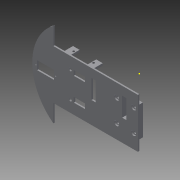
# Autodesk Inventor part: chasis_robot_kedama_rev7
Saved by Autodesk Inventor 2015 (Build 190159000, 159)
## iProperties
Created: 2021-04-17
Part Number: chasis_robot_kedama_rev7
Material: Generic
Document SubType Name: Modeling
Designer: 34617
Density: 1 g/cm^3
Appearance: Default
Author: 34617
Autodesk Inventor part; units mm, degrees
ref_plane "YZ Plane" through (0, 0, 0) normal (1, 0, 0) x (0, 1, 0)
ref_plane "XZ Plane" through (0, 0, 0) normal (0, 1, 0) x (-1, 0, 0)
ref_plane "XY Plane" through (0, 0, 0) normal (0, 0, 1) x (1, 0, 0)
sketch "Sketch1" plane through (0, 0, 0) normal (0, 1, 0) x (-1, 0, 0)
  line L0 (0, -60) -> (150, -60) construction
  line L1 (75, 0) -> (75, -120) construction
  line L2 (150, 0) -> (120, 0) construction
  line L3 (120, 0) -> (120, -120) construction
  line L4 (120, -120) -> (150, -120) construction
  arc A0 (120, -120) -> (120, 0) centre (75, -60) ccw
  line L5 (0, -25) -> (120, -25)
  line L6 (120, -25) -> (120, 0)
  line L7 (0, -95) -> (120, -95)
  line L8 (120, -95) -> (120, -120)
  line L9 (0, -25) -> (0, -95)
  point P0 (0, 0)
  dimension "d2" = 30
  dimension "d4" = 120
  dimension "d6" = 120
  dimension "d7" = 75
  dimension "d8" = 60
  dimension "d9" = 95
  dimension "d10" = 25
  dimension "d11" = 0
  dimension "d12" = 120
  dimension "d13" = 30
  dimension "d14" = 30
  dimension "d15" = 0
  dimension "d16" = 120
  constraints: 20 end point, 6 parallel, 2 point on circle, 1 centre point, 1 horizontal, 1 midpoint, 1 perpendicular, 1 tangent, 1 vertical
  measures "d2" distance of L4.end L3.end
  measures "d4" distance of L5.start L5.end
  measures "d6" distance of L7.start L7.end
  measures "d7" radius of A0
  measures "d8" distance between parallel lines of L2 L0
  measures "d9" distance between parallel lines of L2 L7
  measures "d10" distance between parallel lines of L2 L5
  measures "d11" distance from line of point (0, 0) L2
  measures "d12" distance from line of point (0, 0) L6
  measures "d13" distance from line of L2.start L6
  measures "d14" distance from line of L0.end L6
  measures "d15" distance from line of L1.start L2
  measures "d16" distance from line of L0.start L6
extrude "Extrusion1" add sketch "Sketch1" along normal blind 2
sketch "Sketch2" plane through (0, 2, 0) normal (0, 1, 0) x (1, 0, 0)
  line L0 (0, 25) -> (0, 95) construction
  line L1 (0, 60) -> (-150, 60) construction
  arc A0 (-120, 120) -> (-120, 0) centre (-75, 60) ccw construction
  line L2 (-117.4507, 52.0399) -> (-117.4507, 68.4308) construction
  line L3 (-114.9012, 60) -> (-114.9012, 66.1) construction
  line L4 (-114.9012, 66.1) -> (-147.0012, 66.1) construction
  line L5 (-147.0012, 66.1) -> (-147.0012, 53.9) construction
  line L6 (-114.9012, 53.9) -> (-114.9012, 60) construction
  line L7 (-147.0012, 60) -> (-147.0012, 62) construction
  line L8 (-147.0012, 62) -> (-143.0012, 62) construction
  line L9 (-143.0012, 62) -> (-143.0012, 58) construction
  line L10 (-143.0012, 58) -> (-147.0012, 58) construction
  line L11 (-147.0012, 60) -> (-147.0012, 58) construction
  line L12 (-143.0012, 58) -> (-147.0012, 62) construction
  line L13 (-143.0012, 62) -> (-147.0012, 58) construction
  circle A1 centre (-145.0012, 60) radius 1
  line L14 (-114.9012, 60) -> (-114.9012, 62) construction
  line L15 (-114.9012, 62) -> (-118.9012, 62) construction
  line L16 (-118.9012, 62) -> (-118.9012, 58) construction
  line L17 (-118.9012, 58) -> (-114.9012, 58) construction
  line L18 (-118.9012, 62) -> (-114.9012, 62) construction
  line L19 (-114.9012, 58) -> (-114.9012, 62) construction
  line L20 (-114.9012, 58) -> (-118.9012, 62) construction
  line L21 (-114.9012, 62) -> (-118.9012, 58) construction
  circle A2 centre (-116.9012, 60) radius 1
  line L22 (-145.0012, 60) -> (-116.9012, 60) construction
  line L23 (-143.0012, 66.0861) -> (-118.9012, 66.1)
  line L24 (-118.9012, 66.1) -> (-118.8942, 54)
  line L25 (-118.8942, 54) -> (-142.9942, 54)
  line L26 (-142.9942, 54) -> (-142.9942, 66.1)
  point P0 (0, 0)
  dimension "d22" = 117.4507
  dimension "d103" = 32.1
  dimension "d104" = 12.2
  dimension "d105" = 32.1
  dimension "d106" = 2
  dimension "d107" = 4
  dimension "d108" = 4
  dimension "d109" = 2
  dimension "d113" = 2
  dimension "d114" = 28.1
  dimension "d116" = 114.9012
  dimension "d117" = 2
  dimension "d118" = 118.9012
  dimension "d119" = 8.4308
  dimension "d120" = 7.9601
  dimension "d124" = 24.1
  dimension "d125" = 12.1
  dimension "d127" = 0.033
  dimension "d128" = 24.1
  dimension "d129" = 12.1
  constraints: 52 end point, 11 perpendicular, 11 point on line, 4 collinear, 4 midpoint, 2 centre point, 2 parallel, 1 horizontal, 1 point on circle
  measures "d22" distance between parallel lines of L2 L0
  measures "d103" distance of L3.end L4.end
  measures "d104" distance of L4.end L5.end
  measures "d105" distance of L5.end L6.start
  measures "d106" distance of L7.start L7.end
  measures "d107" distance of L7.end L8.end
  measures "d108" distance of L8.end L9.end
  measures "d109" diameter of A1
  measures "d113" diameter of A2
  measures "d114" distance of L22.start L22.end
  measures "d116" distance between parallel lines of L3 L0
  measures "d117" distance between parallel lines of L1 L15
  measures "d118" distance from line of L0.end L16
  measures "d119" distance from line of L2.end L1
  measures "d120" distance from line of L2.start L1
  measures "d124" distance of L23.start L23.end
  measures "d125" distance of L23.end L24.end
  measures "d127" angle of L24 L0
  measures "d128" distance of L24.end L25.end
  measures "d129" distance of L25.end L26.end
sketch "Sketch3" plane through (0, 2, 0) normal (0, 1, 0) x (1, 0, 0)
  line L0 (0, 25) -> (0, 95) construction
  line L1 (0, 60) -> (-150, 60) construction
  circle A0 centre (-30.0032, 43.5012) radius 2
  circle A1 centre (-30.0032, 75.0012) radius 2
  circle A2 centre (-6.0032, 75.0012) radius 2
  circle A3 centre (-6.0032, 43.5012) radius 2
  line L2 (-30.0032, 43.5012) -> (-30.0032, 75.0012) construction
  line L3 (-6.0032, 43.5012) -> (-6.0032, 75.0012) construction
  line L4 (-30.0032, 43.5012) -> (-6.0032, 43.5012) construction
  line L5 (-30.0032, 75.0012) -> (-6.0032, 75.0012) construction
  point P0 (0, 0)
  dimension "d29" = 150
  dimension "d36" = 4
  dimension "d37" = 4
  dimension "d41" = 31.5
  dimension "d42" = 31.5
  dimension "d43" = 24
  dimension "d44" = 24
  dimension "d45" = 6.0032
  dimension "d46" = 16.4988
  constraints: 10 end point, 4 centre point, 2 equal radius, 2 horizontal, 2 vertical, 1 midpoint
  measures "d29" distance of L1.start L1.end
  measures "d36" diameter of A0
  measures "d37" diameter of A1
  measures "d41" distance of L2.start L2.end
  measures "d42" distance of L3.start L3.end
  measures "d43" distance of L2.start L3.start
  measures "d44" distance of L2.end L3.end
  measures "d45" distance between parallel lines of L0 L3
  measures "d46" distance between parallel lines of L1 L4
extrude "Extrusion3" cut sketch "Sketch3" against normal blind 11
sketch "Sketch4" plane through (0, 2, 0) normal (0, 1, 0) x (1, 0, 0)
  line L0 (0, 95) -> (-120, 95) construction
  line L1 (-120, 25) -> (-50, 25) construction
  line L2 (-50, 25) -> (-50, 95) construction
  line L3 (-50, 95) -> (-120, 95) construction
  line L4 (-120, 95) -> (-120, 25) construction
  line L5 (-120, 95) -> (-50, 95) construction
  line L6 (-50, 95) -> (-50, 85) construction
  line L7 (-120, 85) -> (-120, 95) construction
  line L8 (-50, 25) -> (-50, 35) construction
  line L9 (-120, 35) -> (-120, 25) construction
  line L10 (-120, 30) -> (-50, 30) construction
  line L11 (-75, 80) -> (-91, 80)
  line L12 (-91, 40) -> (-75, 40)
  line L13 (-85, 95) -> (-85, 73) construction
  line L14 (-91, 73) -> (-75, 73)
  line L15 (-75, 73) -> (-75, 80) construction
  line L16 (-91, 80) -> (-91, 73)
  line L17 (-75, 80) -> (-75, 73)
  line L18 (-75, 73) -> (-75, 25) construction
  line L19 (-91, 47) -> (-75, 47)
  line L20 (-91, 47) -> (-91, 40)
  line L21 (-75, 47) -> (-75, 40)
  line L22 (-85, 73) -> (-85, 25) construction
  line L23 (-75, 80) -> (-75, 95) construction
  line L24 (-91, 80) -> (-91, 95) construction
  line L25 (-85, 95) -> (-91, 95)
  line L26 (-91, 95) -> (-91, 92.5)
  line L27 (-91, 92.5) -> (-79, 92.5)
  line L28 (-79, 92.5) -> (-79, 95)
  line L29 (-85, 25) -> (-91, 25)
  line L30 (-120, 25) -> (0, 25) projected
  line L31 (-91, 25) -> (-91, 27.5)
  line L32 (-91, 27.5) -> (-79, 27.5)
  line L33 (-79, 27.5) -> (-79, 25)
  line L34 (-85, 25) -> (-79, 25)
  line L35 (-79, 27.5) -> (-91, 27.5)
  line L36 (-75, 40) -> (-70, 40)
  line L37 (-70, 40) -> (-70, 47)
  line L38 (-70, 47) -> (-75, 47)
  line L39 (-75, 73) -> (-69.9974, 73)
  line L40 (-69.9974, 73) -> (-69.9974, 80)
  line L41 (-69.9974, 80) -> (-75, 80)
  point P0 (0, 0)
  dimension "d49" = 70
  dimension "d51" = 10
  dimension "d52" = 10
  dimension "d70" = 6
  dimension "d71" = 2.5
  dimension "d72" = 12
  dimension "d73" = 6
  dimension "d74" = 2.5
  dimension "d75" = 12
  dimension "d76" = 55
  dimension "d77" = 22
  dimension "d78" = 65
  dimension "d79" = 0
  dimension "d80" = 25
  dimension "d81" = 70
  dimension "d219" = 5
  dimension "d220" = 7
  dimension "d221" = 16
  dimension "d222" = 16
  constraints: 80 end point, 17 perpendicular, 11 parallel, 8 point on line, 4 collinear, 3 horizontal, 3 midpoint, 1 vertical
  measures "d49" distance of L3.end L2.end
  measures "d51" distance of L5.end L6.end
  measures "d52" distance of L8.start L8.end
  measures "d70" distance of L13.start L25.end
  measures "d71" distance of L25.end L26.end
  measures "d72" distance of L26.end L27.end
  measures "d73" distance of L22.end L29.end
  measures "d74" distance of L29.end L31.end
  measures "d75" distance of L31.end L32.end
  measures "d76" distance between parallel lines of L30 L11
  measures "d77" distance between parallel lines of L30 L19
  measures "d78" distance between parallel lines of L10 L0
  measures "d79" distance between parallel lines of L2 L6
  measures "d80" distance between parallel lines of L18 L6
  measures "d81" distance from line of L18.end L0
  measures "d219" distance of L12.end L36.end
  measures "d220" distance of L39.end L40.end
  measures "d221" distance of L12.start L12.end
  measures "d222" distance of L14.start L14.end
extrude "Extrusion5" cut sketch "Sketch4" against normal blind 3 contours L17 L14 L16 L11 | L20 L19 L21 L12
sketch "Sketch5" plane through (0, 2, 0) normal (0, 1, 0) x (1, 0, 0)
  line L0 (-120, 25) -> (0, 25) construction
  line L1 (-85, 25) -> (-85, 95) construction
  line L2 (0, 95) -> (-120, 95) construction
  line L3 (-85, 25) -> (-91, 25)
  line L4 (-85, 25) -> (-79, 25)
  line L5 (-85, 95) -> (-91, 95)
  line L6 (-85, 95) -> (-79, 95)
  line L7 (-85, 28) -> (-101.1, 28)
  line L8 (-85, 28) -> (-68.9, 28)
  line L9 (-85, 92) -> (-101.1, 92)
  line L10 (-85, 92) -> (-68.9, 92)
  line L11 (-68.9, 92) -> (-68.9, 95)
  line L12 (0, 95) -> (-120, 95) projected
  line L13 (-101.1, 92) -> (-101.1, 95)
  line L14 (-68.9, 95) -> (-101.1, 95)
  line L15 (-101.1, 28) -> (-101.1, 25)
  line L16 (-68.9, 25) -> (-101.1, 25)
  line L17 (-68.9, 28) -> (-68.9, 25)
  point P0 (0, 0)
  dimension "d84" = 6
  dimension "d157" = 16.1
  dimension "d158" = 16.1
  dimension "d159" = 16.1
  dimension "d160" = 16.1
  dimension "d169" = 90
  dimension "d170" = 90
  dimension "d171" = 67
  dimension "d172" = 3
  dimension "d173" = 0
  dimension "d174" = 16.1
  dimension "d175" = 68.9
  dimension "d176" = 10.1
  dimension "d177" = 10.1
  dimension "d178" = 22.1
  constraints: 30 end point, 10 point on line, 5 perpendicular, 3 collinear, 2 horizontal, 1 vertical
  measures "d84" distance of L1.start L3.end
  measures "d157" distance of L7.start L7.end
  measures "d158" distance of L7.start L8.end
  measures "d159" distance of L9.start L9.end
  measures "d160" distance of L9.start L10.end
  measures "d169" angle of L9 L11
  measures "d170" angle of L7 L11
  measures "d171" distance between parallel lines of L12 L8
  measures "d172" distance between parallel lines of L10 L2
  measures "d173" distance between parallel lines of L11 L17
  measures "d174" distance between parallel lines of L11 L1
  measures "d175" distance from line of L2.start L11
  measures "d176" distance from line of L6.end L11
  measures "d177" distance from line of L4.end L11
  measures "d178" distance from line of L5.end L11
extrude "Extrusion6" add sketch "Sketch5" along normal blind 12
sketch "Sketch6" plane through (-120, 0, -25) normal (0, 0, 1) x (1, 0, 0)
  line L0 (120, 0) -> (0, 0) construction
  line L1 (18.9, 2) -> (51.1, 2) construction
  line L2 (18.9, 2) -> (18.9, 14) construction
  line L3 (18.9, 8) -> (51.1, 8) construction
  line L4 (51.1, 2) -> (51.1, 14) construction
  line L5 (18.9, 8) -> (19.4, 8) construction
  line L6 (19.4, 8) -> (19.4, 14) construction
  line L7 (19.4, 8) -> (19.4, 2) construction
  line L8 (51.1, 2) -> (18.9, 2) construction
  line L9 (51.1, 8) -> (50.6, 8) construction
  line L10 (50.6, 8) -> (50.6, 14) construction
  line L11 (50.6, 14) -> (50.6, 2) construction
  line L12 (19.4, 8) -> (20.9, 8) construction
  circle A0 centre (20.9, 8) radius 1.5
  line L13 (50.6, 8) -> (49.1, 8) construction
  circle A1 centre (49.1, 8) radius 1.5
  dimension "d162" = 0.5
  dimension "d163" = 0.5
  dimension "d164" = 1.5
  dimension "d165" = 3
  dimension "d166" = 1.5
  dimension "d167" = 3
  dimension "d168" = 32.2
  dimension "d179" = 14
  dimension "d180" = 14
  constraints: 20 end point, 8 point on line, 2 centre point, 2 coincident, 2 midpoint, 2 perpendicular, 1 horizontal
  measures "d162" distance of L3.start L5.end
  measures "d163" distance of L3.end L9.end
  measures "d164" distance of L5.end L12.end
  measures "d165" diameter of A0
  measures "d166" distance of L9.end L13.end
  measures "d167" diameter of A1
  measures "d168" distance of L3.start L3.end
  measures "d179" distance from line of L10.end L0
  measures "d180" distance from line of L6.end L0
extrude "Extrusion7" cut sketch "Sketch6" against normal blind 3
sketch "Sketch7" plane through (0, 0, -95) normal (0, 0, -1) x (-1, 0, 0)
  line L0 (120, 0) -> (0, 0) construction
  line L1 (68.9, 2) -> (101.1, 2) construction
  line L2 (68.9, 2) -> (101.1, 2) construction
  line L3 (68.9, 2) -> (68.9, 14) construction
  line L4 (68.9, 8) -> (101.1, 8) construction
  circle A0 centre (70.9, 8) radius 1.5 projected
  circle A1 centre (70.9, 8) radius 1.5
  circle A2 centre (99.1, 8) radius 1.5 projected
  circle A3 centre (99.1, 8) radius 1.5
  constraints: 4 end point, 2 centre point, 2 coincident, 1 collinear, 1 horizontal, 1 midpoint
extrude "Extrusion8" cut sketch "Sketch7" against normal blind 3
extrude "Extrusion9" cut sketch "Sketch2" against normal blind 3 contours A1 | A2
sketch "Sketch9" plane through (0, 2, 0) normal (0, 1, 0) x (1, 0, 0)
  circle A0 centre (-116.9012, 60) radius 1 construction
  circle A1 centre (-145.0012, 60) radius 1 construction
  line L0 (-116.9012, 60) -> (-145.0012, 60) construction
  line L1 (-145.0012, 60) -> (-150, 60) construction
  arc A2 (-120, 120) -> (-120, 0) centre (-75, 60) ccw construction
  line L2 (-144.0012, 60) -> (-143.0012, 60) construction
  line L3 (-143.0012, 60) -> (-143.0012, 66.1)
  line L4 (-143.0012, 66.1) -> (-119.0012, 66.1)
  line L5 (-119.0012, 66.1) -> (-119.0012, 53.9)
  line L6 (-119.0012, 53.9) -> (-143.0012, 53.9)
  line L7 (-143.0012, 53.9) -> (-143.0012, 60)
  point P0 (0, 0)
  dimension "d130" = 1
  dimension "d131" = 6.1
  dimension "d132" = 24
  dimension "d133" = 12.2
  constraints: 16 end point, 5 perpendicular, 4 point on line, 1 horizontal, 1 horizontal alignment, 1 point on circle, 1 other
  measures "d130" distance of L2.start L2.end
  measures "d131" distance of L2.end L3.end
  measures "d132" distance of L3.end L4.end
  measures "d133" distance of L4.end L5.end
extrude "Extrusion10" cut sketch "Sketch9" against normal blind 2
sketch "Sketch10" plane through (0, 2, 0) normal (0, 1, 0) x (1, 0, 0)
  line L0 (0, 25) -> (0, 95) projected
  line L1 (-34.3549, 37.8531) -> (0, 37.8531)
  line L2 (0, 37.8531) -> (0, 80.7294)
  line L3 (0, 80.7294) -> (-34.3549, 80.7294)
  line L4 (-34.3549, 80.7294) -> (-34.3549, 37.8531)
  circle A0 centre (-30.0032, 43.5012) radius 2 projected
  circle A1 centre (-30.0032, 43.5012) radius 2
  circle A2 centre (-30.0032, 75.0012) radius 2 projected
  circle A3 centre (-30.0032, 75.0012) radius 2
  circle A4 centre (-6.0032, 43.5012) radius 2 projected
  circle A5 centre (-6.0032, 43.5012) radius 2
  circle A6 centre (-6.0032, 75.0012) radius 2.1402
  point P0 (0, 0)
  dimension "d136" = 34.3548
  dimension "d137" = 42.8763
  dimension "d138" = 14.2706
  dimension "d147" = 4.2805
  dimension "d148" = 4
  dimension "d149" = 4
  dimension "d150" = 4
  dimension "d151" = 6.0032
  dimension "d152" = 5.7282
  constraints: 8 end point, 4 centre point, 3 coincident, 2 parallel, 1 horizontal, 1 perpendicular, 1 point on line
  measures "d136" distance between parallel lines of L4 L0
  measures "d137" distance between parallel lines of L3 L1
  measures "d138" distance from line of L0.end L3
  measures "d147" diameter of A6
  measures "d148" diameter of A5
  measures "d149" diameter of A3
  measures "d150" diameter of A1
  measures "d151" distance from line of A6.centre L0
  measures "d152" distance from line of A6.centre L3
extrude "Extrusion11" add sketch "Sketch10" along normal blind 5 contours L1 L4 L3 L0 | A0 | A2 | A4 | A6
sketch "Sketch11" plane through (0, 7, 0) normal (0, 1, 0) x (1, 0, 0)
  circle A0 centre (-30.0032, 43.5012) radius 2 projected
  circle A1 centre (-30.0032, 43.5012) radius 2
  circle A2 centre (-30.0032, 75.0012) radius 2 projected
  circle A3 centre (-30.0032, 75.0012) radius 2
  circle A4 centre (-6.0032, 43.5012) radius 2 projected
  circle A5 centre (-6.0032, 43.5012) radius 2
  circle A6 centre (-6.0032, 75.0012) radius 2 projected
  circle A7 centre (-6.0032, 75.0012) radius 2
  point P0 (0, 0)
  constraints: 4 centre point, 4 coincident
extrude "Extrusion12" cut sketch "Sketch11" against normal blind 11
sketch "Sketch13" plane through (0, 2, 0) normal (0, 1, 0) x (1, 0, 0)
  point P0 (0, 0)
sketch "Sketch14" plane through (0, 2, 0) normal (0, 1, 0) x (1, 0, 0)
  line L0 (-122.4098, 34.6229) -> (-134.4098, 34.6229)
  line L1 (-134.4098, 34.6229) -> (-134.4098, 42.6229)
  line L2 (-134.4098, 42.6229) -> (-122.4098, 42.6229)
  line L3 (-122.4098, 42.6229) -> (-122.4098, 34.6229)
  point P0 (0, 0)
  dimension "d183" = 12
  dimension "d184" = 8
  constraints: 8 end point, 2 parallel, 1 horizontal, 1 perpendicular
  measures "d183" distance of L1.end L2.end
  measures "d184" distance of L0.end L1.end
extrude "Extrusion14" add sketch "Sketch14" along normal blind 0.5
sketch "Sketch16" plane through (0, 2.5, 0) normal (0, 1, 0) x (1, 0, 0)
  line L0 (-130.4881, 40.8759) -> (-125.3198, 40.8759) construction
  line L1 (-125.3198, 40.8759) -> (-125.3198, 24.6109) construction
  line L2 (-125.3198, 24.6109) -> (-130.4881, 24.6109) construction
  line L3 (-130.4881, 24.6109) -> (-130.4881, 40.8759) construction
  line L4 (-123.6414, 30.8759) -> (-125.3675, 30.8759)
  line L5 (-125.3675, 30.8759) -> (-129.0223, 35.5274)
  line L6 (-129.0223, 35.5274) -> (-129.6057, 34.871)
  line L7 (-129.6057, 34.871) -> (-129.6057, 30.8759)
  line L8 (-129.6057, 30.8759) -> (-130.9347, 30.8759)
  line L9 (-130.9347, 30.8759) -> (-130.9347, 40.8759)
  line L10 (-130.9347, 40.8759) -> (-129.6057, 40.8759)
  line L11 (-129.6057, 40.8759) -> (-129.6057, 36.2811)
  line L12 (-129.6057, 36.2811) -> (-125.5052, 40.8759)
  line L13 (-125.5052, 40.8759) -> (-123.8845, 40.8759)
  line L14 (-123.8845, 40.8759) -> (-128.0255, 36.4107)
  line L15 (-128.0255, 36.4107) -> (-123.6414, 30.8759)
  point P0 (0, 0)
  dimension "d270" = 5.1682
  dimension "d271" = 16.265
  dimension "d272" = 125.3198
  dimension "d273" = 40.8759
  constraints: 1 horizontal, 2 other
  measures "d270" distance between parallel lines of L3 L1
  measures "d271" distance between parallel lines of L0 L2
  measures "d272" distance from line of point (0, 0) L1
  measures "d273" distance from line of point (0, 0) L0
extrude "Extrusion15" add sketch "Sketch16" along normal blind 1.5
sketch "Sketch17" plane through (-120, 0, -25) normal (0, 0, 1) x (1, 0, 0)
  line L0 (18.9, 14) -> (51.1, 14) projected
  line L1 (23.2569, 14) -> (46.8571, 14)
  line L2 (46.8571, 14) -> (46.8571, 2)
  line L3 (46.8571, 2) -> (23.2569, 2)
  line L4 (23.2569, 2) -> (23.2569, 14)
  point P0 (120, 0)
  dimension "d189" = 12
  dimension "d190" = 23.6002
  dimension "d191" = 73.1429
  constraints: 8 end point, 2 parallel, 1 horizontal, 1 perpendicular, 1 point on line
  measures "d189" distance of L3.end L1.start
  measures "d190" distance of L2.end L3.end
  measures "d191" distance from line of point (120, 0) L2
extrude "Extrusion16" cut sketch "Sketch17" against normal blind 3
sketch "Sketch18" plane through (-120, 0, -25) normal (0, 0, 1) x (1, 0, 0)
  line L0 (18.9, 2) -> (13.9, 2)
  line L1 (13.9, 2) -> (13.9, 14)
  line L2 (13.9, 14) -> (18.9, 14)
  line L3 (18.9, 14) -> (18.9, 2)
  line L4 (51.1, 2) -> (56.1, 2)
  line L5 (56.1, 2) -> (56.1, 14)
  line L6 (56.1, 14) -> (51.1, 14)
  line L7 (51.1, 14) -> (51.1, 2)
  point P0 (120, 0)
  dimension "d194" = 5
  dimension "d195" = 12
  dimension "d196" = 5
  dimension "d197" = 12
  constraints: 16 end point, 4 parallel, 2 horizontal, 2 perpendicular
  measures "d194" distance of L1.end L2.end
  measures "d195" distance of L0.end L1.end
  measures "d196" distance of L6.end L5.end
  measures "d197" distance of L4.end L5.end
extrude "Extrusion17" add sketch "Sketch18" against normal blind 3
sketch "Sketch19" plane through (0, 0, -95) normal (0, 0, -1) x (-1, 0, 0)
  line L0 (73.1429, 14) -> (96.7431, 14)
  line L1 (96.7431, 14) -> (96.7431, 2)
  line L2 (96.7431, 2) -> (73.1429, 2)
  line L3 (73.1429, 2) -> (73.1429, 14)
  point P0 (0, 0)
  constraints: 8 end point, 2 parallel, 1 horizontal, 1 perpendicular
extrude "Extrusion18" cut sketch "Sketch19" against normal blind 3
sketch "Sketch20" plane through (0, 0, -95) normal (0, 0, -1) x (-1, 0, 0)
  line L0 (68.9, 2) -> (63.9, 2)
  line L1 (63.9, 2) -> (63.9, 14)
  line L2 (63.9, 14) -> (68.9, 14)
  line L3 (68.9, 14) -> (68.9, 2)
  line L4 (101.1, 2) -> (106.1, 2)
  line L5 (106.1, 2) -> (106.1, 14)
  line L6 (106.1, 14) -> (101.1, 14)
  line L7 (101.1, 14) -> (101.1, 2)
  point P0 (0, 0)
  constraints: 16 end point, 4 parallel, 2 horizontal, 2 perpendicular
extrude "Extrusion19" add sketch "Sketch20" against normal blind 3
sketch "Sketch21" plane through (0, 0, 0) normal (0, -1, 0) x (1, 0, 0)
  circle A0 centre (-6.036, -74.9232) radius 3.5
  circle A1 centre (-30.0796, -74.9232) radius 3.5
  circle A2 centre (-30.0796, -43.3906) radius 3.5
  circle A3 centre (-6.036, -43.3906) radius 3.5
  point P0 (0, 0)
  dimension "d204" = 7
  dimension "d205" = 7
  dimension "d206" = 7
  dimension "d207" = 7
  constraints: 4 centre point
  measures "d204" diameter of A0
  measures "d205" diameter of A1
  measures "d206" diameter of A2
  measures "d207" diameter of A3
extrude "Extrusion20" cut sketch "Sketch21" against normal blind 2
sketch "Sketch22" plane through (0, 2, 0) normal (0, 1, 0) x (1, 0, 0)
  line L0 (-78.4615, 36.6997) -> (-113.3615, 36.6997) construction
  line L1 (-113.3615, 36.6997) -> (-113.3615, 83.9997) construction
  line L2 (-113.3615, 83.9997) -> (-78.4615, 83.9997) construction
  line L3 (-78.4615, 83.9997) -> (-78.4615, 36.6997) construction
  line L4 (-78.4615, 60.3497) -> (-113.3615, 60.3497) construction
  circle A0 centre (-95.9115, 41.8497) radius 2
  circle A1 centre (-95.9115, 78.8497) radius 2
  line L5 (-17.2206, 25.8993) -> (-68.7206, 25.8993) construction
  line L6 (-68.7206, 25.8993) -> (-68.7206, 93.3993) construction
  line L7 (-68.7206, 93.3993) -> (-17.2206, 93.3993) construction
  line L8 (-17.2206, 93.3993) -> (-17.2206, 25.8993) construction
  line L9 (-68.7206, 93.3993) -> (-62.4206, 93.3993) construction
  line L10 (-62.4206, 93.3993) -> (-62.4206, 56.4993) construction
  line L11 (-62.4206, 56.4993) -> (-68.7206, 56.4993) construction
  line L12 (-68.7206, 56.4993) -> (-67.2206, 56.4993) construction
  line L13 (-67.2206, 56.4993) -> (-61.2206, 56.4993)
  line L14 (-61.2206, 56.4993) -> (-61.2206, 83.4993)
  line L15 (-67.2206, 56.4993) -> (-67.2206, 83.4993)
  line L16 (-67.2206, 83.4993) -> (-61.2206, 83.4993)
  line L17 (-17.2206, 83.4993) -> (-61.2206, 83.4993) construction
  line L18 (-18.6258, 83.4993) -> (-24.6258, 83.4993)
  line L19 (-24.6258, 83.4993) -> (-24.6258, 56.4993)
  line L20 (-24.6258, 56.4993) -> (-18.6258, 56.4993)
  line L21 (-18.6258, 56.4993) -> (-18.6258, 83.4993)
  point P0 (0, 0)
  dimension "d210" = 34.9
  dimension "d211" = 47.3
  dimension "d213" = 4
  dimension "d215" = 4
  dimension "d216" = 37
  dimension "d223" = 67.5
  dimension "d224" = 51.5
  dimension "d225" = 6.3
  dimension "d226" = 36.9
  dimension "d227" = 1.5
  dimension "d228" = 6
  dimension "d229" = 27
  dimension "d236" = 27
  dimension "d237" = 6
  dimension "d238" = 1.4052
  dimension "d239" = 61.2409
  dimension "d240" = 0.5004
  dimension "d241" = 17.2206
  dimension "d242" = 83.4993
  dimension "d243" = 78.6909
  dimension "d244" = 4.6495
  dimension "d245" = 78.6909
  constraints: 44 end point, 7 perpendicular, 6 parallel, 6 point on line, 3 horizontal, 2 centre point, 2 midpoint, 2 vertical
  measures "d210" distance of L0.start L0.end
  measures "d211" distance of L2.end L0.start
  measures "d213" diameter of A0
  measures "d215" diameter of A1
  measures "d216" distance of A1.centre A0.centre
  measures "d223" distance of L5.end L6.end
  measures "d224" distance of L5.start L5.end
  measures "d225" distance of L6.end L9.end
  measures "d226" distance of L9.end L10.end
  measures "d227" distance of L11.end L12.end
  measures "d228" distance of L12.end L13.end
  measures "d229" distance of L13.end L14.end
  measures "d236" distance of L18.end L19.end
  measures "d237" distance of L18.start L18.end
  measures "d238" distance between parallel lines of L8 L21
  measures "d239" distance between parallel lines of L8 L3
  measures "d240" distance between parallel lines of L2 L17
  measures "d241" distance from line of point (0, 0) L8
  measures "d242" distance from line of point (0, 0) L17
  measures "d243" distance from line of A1.centre L8
  measures "d244" distance from line of A1.centre L18
  measures "d245" distance from line of A0.centre L8
extrude "Extrusion21" cut sketch "Sketch22" against normal blind 3 contours A0 | A1
sketch "Sketch23" plane through (0, 0, 0) normal (0, -1, 0) x (1, 0, 0)
  line L0 (-19.3168, -94.1992) -> (-67.4168, -94.1992) construction
  line L1 (-67.4168, -94.1992) -> (-67.4168, -26.6992) construction
  line L2 (-67.4168, -26.6992) -> (-19.3168, -26.6992) construction
  line L3 (-19.3168, -26.6992) -> (-19.3168, -94.1992) construction
  line L4 (-67.4168, -26.6992) -> (-65.9168, -26.6992) construction
  line L5 (-65.9168, -26.6992) -> (-65.9168, -64.1992) construction
  line L6 (-65.9168, -64.1992) -> (-59.9168, -64.1992)
  line L7 (-59.9168, -64.1992) -> (-59.9168, -37.1992)
  line L8 (-59.9168, -37.1992) -> (-65.9168, -37.1992)
  line L9 (-65.9168, -37.1992) -> (-65.9168, -64.1992)
  line L10 (-59.9168, -64.1992) -> (-19.3168, -64.1992) construction
  line L11 (-19.3168, -37.1992) -> (-21.5168, -37.1992) construction
  line L12 (-59.9168, -37.1992) -> (-22.4168, -37.1992) construction
  line L13 (-22.4168, -37.1992) -> (-16.4168, -37.1992)
  line L14 (-63.9, -25) -> (0, -25) construction
  line L15 (-22.4168, -37.1992) -> (-22.4168, -64.1992)
  line L16 (-22.4168, -64.1992) -> (-16.4168, -64.1992)
  line L17 (-16.4168, -64.1992) -> (-16.4168, -37.1992)
  point P0 (0, 0)
  dimension "d248" = 67.5
  dimension "d249" = 48.1
  dimension "d250" = 1.5
  dimension "d251" = 37.5
  dimension "d252" = 6
  dimension "d253" = 27
  dimension "d254" = 6
  dimension "d260" = 37.5
  dimension "d261" = 6
  dimension "d262" = 6
  dimension "d263" = 90
  dimension "d264" = 12.1992
  dimension "d265" = 16.4168
  dimension "d266" = 37.1992
  dimension "d267" = 5.1
  constraints: 34 end point, 6 perpendicular, 6 point on line, 3 parallel, 2 horizontal, 1 collinear
  measures "d248" distance of L0.end L1.end
  measures "d249" distance of L1.end L2.end
  measures "d250" distance of L1.end L4.end
  measures "d251" distance of L4.end L5.end
  measures "d252" distance of L5.end L6.end
  measures "d253" distance of L6.end L7.end
  measures "d254" distance of L7.end L8.end
  measures "d260" distance of L7.end L12.end
  measures "d261" distance of L12.end L13.end
  measures "d262" distance of L15.end L16.end
  measures "d263" angle of L11 L17
  measures "d264" distance between parallel lines of L14 L12
  measures "d265" distance from line of point (0, 0) L17
  measures "d266" distance from line of point (0, 0) L11
  measures "d267" distance from line of L11.end L17
extrude "Extrusion22" cut sketch "Sketch23" against normal blind 8
body "Solid1"
